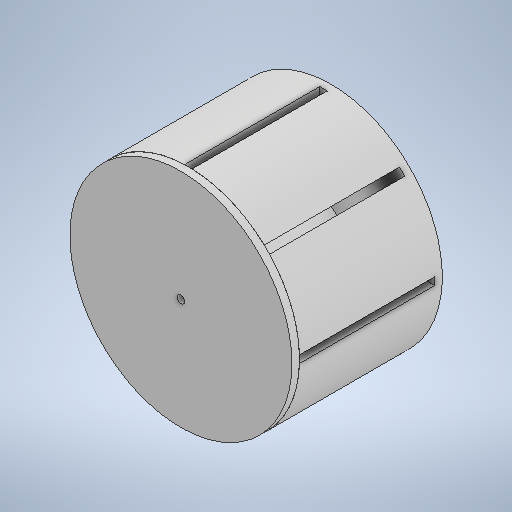
# Autodesk Inventor part: Part26
Saved by Autodesk Inventor 2025.1 (Build 291241020, 241B)
## iProperties
Created: 2024-11-27
Part Number: Part26
Material: Generic
Document SubType Name: Modeling
Designer: User
Density: 1 g/cm^3
Appearance: Default
Author: User
Autodesk Inventor part; units mm, degrees
ref_plane "YZ Plane" through (0, 0, 0) normal (1, 0, 0) x (0, 1, 0)
ref_plane "XZ Plane" through (0, 0, 0) normal (0, 1, 0) x (-1, 0, 0)
ref_plane "XY Plane" through (0, 0, 0) normal (0, 0, 1) x (1, 0, 0)
sketch "Sketch1" plane through (0, 0, 0) normal (0, 0, 1) x (1, 0, 0)
  point P0 (0, 0)
sketch "Sketch2" plane through (0, 0, 0) normal (0, 0, 1) x (1, 0, 0)
  circle A0 centre (0, 0) radius 10
  line L0 (2.4793, 73.9585) -> (2.4781, 9.6881)
  line L1 (-2.5359, 9.6731) -> (-2.5218, 9.6731)
  line L2 (-2.5218, 9.6768) -> (-2.5207, 73.9571)
  line L3 (-2.4922, 73.958) -> (2.4781, 9.6881) construction
  line L4 (2.4804, 74.3269) -> (-2.5218, 9.6731) construction
  line L5 (-2.5218, 9.6731) -> (-2.5218, 9.6723)
  line L6 (9.283, 2.5) -> (74.717, 2.5)
  line L7 (74.717, 2.5) -> (74.717, -2.5)
  line L8 (74.717, -2.5) -> (9.283, -2.5)
  line L9 (9.283, -2.5) -> (9.283, 2.5)
  line L10 (9.283, 2.5) -> (74.717, -2.5) construction
  line L11 (74.717, 2.5) -> (9.283, -2.5) construction
  line L12 (2.4778, -7.9438) -> (2.5, -7.9438)
  line L13 (2.5, -9.6825) -> (2.5, -73.9578)
  line L14 (2.5, -76.0562) -> (2.4766, -76.0562)
  line L15 (-2.5, -73.9578) -> (-2.5, -9.6825)
  line L16 (-2.5, -7.9438) -> (2.5, -76.0562) construction
  line L17 (2.5, -7.9438) -> (-2.5, -76.0562) construction
  line L18 (-73.9602, 2.427) -> (-9.701, 2.427)
  line L19 (-8.7479, -2.5) -> (-8.7479, -2.573)
  line L20 (-9.6633, -2.573) -> (-73.9553, -2.573)
  line L21 (-75.2519, -2.573) -> (-75.2519, -2.5)
  line L22 (-75.2519, 2.427) -> (-8.7479, -2.573) construction
  line L23 (-8.7479, 2.427) -> (-75.2519, -2.573) construction
  line L24 (50.5283, 54.0638) -> (5.0788, 8.6143)
  line L25 (-1.7678, 1.7678) -> (1.7678, -1.7678)
  line L26 (8.6143, 5.0788) -> (54.0638, 50.5283)
  line L27 (53.4417, 51.1858) -> (5.5504, 8.3182) construction
  line L28 (39.6303, -7.8699) -> (34.6303, 82.4585) construction
  line L29 (-54.0638, -50.5283) -> (-8.6143, -5.0788)
  line L30 (-1.7678, 1.7678) -> (1.7678, -1.7678)
  line L31 (-5.0788, -8.6143) -> (-50.5283, -54.0638)
  line L32 (-51.9756, -52.6739) -> (-8.4008, -5.4246) construction
  line L33 (-52.6739, -51.9756) -> (-5.4246, -8.4008) construction
  arc A1 (73.9597, 2.4421) -> (53.4417, 51.1858) centre (0, 0) ccw
  arc A2 (50.5283, 54.0638) -> (2.452, 73.9594) centre (0, 0) ccw
  arc A3 (-73.9586, -2.4757) -> (-54.0638, -50.5283) centre (0, 0) ccw
  arc A4 (-50.5283, -54.0638) -> (-2.3463, -73.9628) centre (0, 0) ccw
  line L34 (-50.5283, 54.0638) -> (-5.0788, 8.6143)
  line L35 (1.7678, 1.7678) -> (0, 0)
  line L36 (-8.6143, 5.0788) -> (-54.0638, 50.5283)
  line L37 (-84.1138, 80.5783) -> (-5.4456, 8.3872) construction
  line L38 (-80.5783, 84.1138) -> (-1.7678, -1.7678) construction
  arc A5 (-2.4922, 73.958) -> (-50.5283, 54.0638) centre (0, 0) ccw
  arc A6 (-54.0638, 50.5283) -> (-73.9633, 2.3301) centre (0, 0) ccw
  line L39 (5.0788, -8.6143) -> (50.5283, -54.0638)
  line L40 (79.0888, -76.0562) -> (79.3403, -75.8047)
  line L41 (54.0638, -50.5283) -> (8.6143, -5.0788)
  line L42 (1.7678, 1.7678) -> (75.8047, -79.3403) construction
  line L43 (-1.7678, -1.7678) -> (79.3403, -75.8047) construction
  arc A7 (2.3463, -73.9628) -> (50.5283, -54.0638) centre (0, 0) ccw
  arc A8 (54.0638, -50.5283) -> (73.9597, -2.4421) centre (0, 0) ccw
  point P0 (-0.0207, 42)
  point P1 (-0.0207, 74.3122)
  point P2 (42, 0)
  point P3 (0, -42)
  point P4 (-41.9999, -0.073)
  point P5 (37.1303, 37.2943)
  point P6 (-43.6953, -43.6953)
  point P7 (-41.173, 41.173)
  point P8 (38.7862, -38.7862)
  point P9 (73.9578, -2.5)
  point P10 (73.9578, 2.5)
  dimension "d1" = 20
  dimension "d3" = 5
  dimension "d4" = 65.434
  dimension "d5" = 5
  dimension "d6" = 5
  dimension "d7" = 66.504
  dimension "d8" = 5
  dimension "d9" = 5
  dimension "d10" = 5
  dimension "d11" = 5
  dimension "d12" = 5
  constraints: 88 end point, 23 point on circle, 16 point on line, 15 midpoint, 11 parallel, 8 centre point, 3 coincident, 3 horizontal, 3 perpendicular, 1 vertical, 21 other
  measures "d3" distance of L0.end L1.end
  measures "d4" distance of L7.end L8.end
  measures "d5" distance of L6.end L7.end
  measures "d6" distance of L14.start L17.end
  measures "d7" distance of L19.end L21.start
  measures "d8" distance of L23.start L19.end
  measures "d9" distance of L25.end L25.start
  measures "d10" distance of L30.start L30.end
  measures "d11" distance of L35.start L38.end
  measures "d12" distance of L42.end L40.end
extrude "Extrusion1" add sketch "Sketch2" along normal blind 90 contours A0 L6 L9 L8 | L26 A1 L6 A0 | A0 L0 A2 L24 | A0 L34 A5 L2 | L8 A8 L41 A0 | L39 A7 L13 A0 | A0 L18 A6 L36 | L15 A4 L31 A0 | A0 L29 A3 L20 picked at (2.8651, 0.2554)
sketch "Sketch3" plane through (0, 0, 0) normal (0, 0, -1) x (-1, 0, 0)
  circle A0 centre (0, 0) radius 74
  constraints: 1 centre point, 1 coincident
extrude "Extrusion2" add sketch "Sketch3" along normal blind 5
sketch "Sketch4" plane through (0, 0, 90) normal (0, 0, 1) x (1, 0, 0)
  circle A0 centre (0, 0) radius 73.9097
  constraints: 1 centre point, 1 coincident
extrude "Extrusion3" add sketch "Sketch4" along normal blind 5
sketch "Sketch5" plane through (0, 0, 95) normal (0, 0, 1) x (1, 0, 0)
  circle A0 centre (0, 0) radius 2.5
  dimension "d19" = 5
  constraints: 1 centre point, 1 coincident
  measures "d19" diameter of A0
extrude "Extrusion4" cut sketch "Sketch5" against normal through all
body "Solid1"
